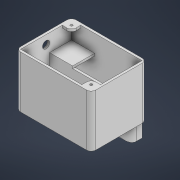
# Autodesk Inventor part: Bike_Telemetry
Saved by Autodesk Inventor 2022 (Build 260153000, 153)
## iProperties
Created: 2022-06-22
Part Number: Bike_Telemetry
Material: Generic
Document SubType Name: Modeling
Designer: Gugarauj07
Density: 1 g/cm^3
Appearance: Default
Author: Gugarauj07
Autodesk Inventor part; units mm, degrees
ref_plane "YZ Plane" through (0, 0, 0) normal (1, 0, 0) x (0, 1, 0)
ref_plane "XZ Plane" through (0, 0, 0) normal (0, 1, 0) x (-1, 0, 0)
ref_plane "XY Plane" through (0, 0, 0) normal (0, 0, 1) x (1, 0, 0)
sketch "Sketch1" plane through (0, 0, 0) normal (0, 0, 1) x (1, 0, 0)
  line L0 (0, 0) -> (65, 0)
  line L1 (65, 0) -> (65, 45)
  line L2 (65, 45) -> (0, 45)
  line L3 (0, 45) -> (0, 0)
  dimension "d3" = 65
  dimension "d4" = 45
  constraints: 8 end point, 2 parallel, 1 horizontal, 1 perpendicular, 1 vertical
  measures "d3" distance of L2.end L1.end
  measures "d4" distance of L1.end L0.end
extrude "Extrusion1" add sketch "Sketch1" along normal blind 48
shell "Shell1" thickness 2 removed faces 1 at (43.3333, 45, 16)
sketch "Sketch2" plane through (2, 2, 2) normal (0, 1, 0) x (1, 0, 0)
  line L0 (61, -44) -> (0, -44) projected
  line L1 (0, -44) -> (10, -44)
  line L2 (10, -44) -> (40, -44)
  line L3 (40, -44) -> (40, -34)
  line L4 (40, -34) -> (10, -34)
  line L5 (10, -34) -> (10, -44)
  line L6 (61, 0) -> (61, -44) projected
  line L7 (0, -44) -> (0, 0) projected
  point P0 (-2, 2)
  dimension "d9" = 30
  dimension "d10" = 10
  dimension "d11" = 61
  dimension "d27" = 10
  constraints: 10 end point, 2 parallel, 1 horizontal, 1 perpendicular, 1 point on line
  measures "d9" distance of L4.end L3.end
  measures "d10" distance of L3.end L2.end
  measures "d11" distance between parallel lines of L6 L7
  measures "d27" distance between parallel lines of L5 L7
extrude "Extrusion2" cut sketch "Sketch2" against normal through all
sketch "Sketch3" plane through (2, 2, 2) normal (0, 1, 0) x (1, 0, 0)
  line L0 (0, 0) -> (0, -44) projected
  line L1 (0, -17) -> (0, 33)
  line L2 (0, -17) -> (44, -17)
  line L3 (44, -17) -> (0, -17)
  line L4 (0, -17) -> (0, -19)
  line L5 (0, -19) -> (44, -19)
  line L6 (44, -19) -> (44, -17)
  point P0 (-2, 2)
  dimension "d16" = 44
  dimension "d17" = 2
  constraints: 12 end point, 2 horizontal, 2 parallel, 2 point on line, 1 collinear, 1 perpendicular
  measures "d16" distance of L1.start L2.end
  measures "d17" distance of L4.end L3.end
extrude "Extrusion3" add sketch "Sketch3" along normal blind 26
fillet "Fillet1" radius 4 1 edges at (0, 22.5, 0)
fillet "Fillet2" radius 4 1 edges at (65, 22.5, 0)
fillet "Fillet3" radius 4 1 edges at (65, 22.5, 48)
fillet "Fillet4" radius 4 1 edges at (0, 22.5, 48)
sketch "Sketch4" plane through (2, 2, 2) normal (1, 0, 0) x (0, 0, -1)
  line L0 (-19, 26) -> (-17, 26) projected
  line L1 (-19, 26) -> (0, 26)
  line L2 (0, 26) -> (0, 28)
  line L3 (0, 28) -> (-19, 28)
  line L4 (-19, 28) -> (-19, 26)
  point P0 (2, -2)
  dimension "d24" = 2
  constraints: 8 end point, 2 parallel, 1 horizontal, 1 perpendicular
  measures "d24" distance of L2.end L1.end
extrude "Extrusion4" add sketch "Sketch4" along normal blind 20
sketch "Sketch8" plane through (2, 2, 2) normal (0, 0, 1) x (1, 0, 0)
  line L0 (0, 43) -> (8, 43)
  line L1 (8, 43) -> (8, 41)
  line L2 (8, 41) -> (0, 41)
  line L3 (0, 41) -> (0, 43)
  point P0 (-2, -2)
  dimension "d28" = 8
  dimension "d29" = 2
  constraints: 8 end point, 2 parallel, 1 horizontal, 1 perpendicular
  measures "d28" distance of L1.end L2.end
  measures "d29" distance of L0.end L1.end
extrude "Extrusion5" add sketch "Sketch8" along normal blind 8
sketch "Sketch10" plane through (4, 45, 0) normal (0, 1, 0) x (1, 0, 0)
  line L0 (6, -2) -> (6, -10) projected
  circle A0 centre (2, -6) radius 1
  point P0 (-4, 0)
  constraints: 1 centre point
extrude "Extrusion7" cut sketch "Sketch10" against normal blind 2
fillet "Fillet6" radius 4 1 edges at (10, 44, 10)
sketch "Sketch13" plane through (63, 45, 46) normal (0, 0, -1) x (-1, 0, 0)
  line L0 (0, -43) -> (0, 0) projected
  line L1 (0, 0) -> (8, 0)
  line L2 (8, 0) -> (8, -2)
  line L3 (8, -2) -> (0, -2)
  line L4 (0, -2) -> (0, 0)
  point P0 (63, -45)
  point P1 (0, -2)
  dimension "d51" = 8
  dimension "d52" = 2
  constraints: 8 end point, 2 parallel, 1 horizontal, 1 perpendicular
  measures "d51" distance of L2.end L3.end
  measures "d52" distance of L1.end L2.end
extrude "Extrusion10" add sketch "Sketch13" along normal blind 8
sketch "Sketch14" plane through (4, 45, 0) normal (0, 1, 0) x (1, 0, 0)
  circle A0 centre (55, -42) radius 1
  point P0 (-4, 0)
  constraints: 1 centre point
extrude "Extrusion11" cut sketch "Sketch14" against normal blind 2
fillet "Fillet7" radius 4 1 edges at (55, 44, 38)
sketch "Sketch15" plane through (4, 0, 0) normal (0, -1, 0) x (1, 0, 0)
  line L0 (57, 0) -> (0, 0)
  line L1 (0, 0) -> (0, 15)
  line L2 (0, 15) -> (57, 15)
  line L3 (57, 15) -> (57, 0)
  constraints: 8 end point, 2 parallel, 1 horizontal, 1 perpendicular
extrude "Extrusion12" add sketch "Sketch15" along normal blind 15
fillet "Fillet8" radius 10 3 edges at (4, -7.5, 15) (61, -7.5, 15) (32.5, -15, 15)
sketch "Sketch16" plane through (0, 0, 0) normal (0, 0, -1) x (-1, 0, 0)
  line L0 (-41, -15) -> (-24, -15)
  line L1 (-24, -15) -> (-24, -10.2203)
  line L2 (-24, -10.2203) -> (-41, -10.2203)
  line L3 (-41, -10.2203) -> (-41, -15)
  point P0 (0, 0)
  point P1 (-4, -15)
  point P2 (-61, -15)
  constraints: 8 end point, 2 parallel, 1 horizontal, 1 perpendicular
extrude "Extrusion13" add sketch "Sketch16" along normal blind 15
fillet "Fillet9" radius 7 2 edges at (41, -12.6102, -15) (24, -12.6102, -15)
sketch "Sketch17" plane through (24, -10.2203, 0) normal (0, 1, 0) x (1, 0, 0)
  line L0 (0, 0) -> (8.5, 0)
  circle A0 centre (8.5, 7.5) radius 4
  point P0 (-24, 0)
  constraints: 2 end point, 1 centre point, 1 horizontal
extrude "Extrusion14" cut sketch "Sketch17" against normal through all
sketch "Sketch19" plane through (2, 2, 46) normal (1, 0, 0) x (0, 0, -1)
  circle A0 centre (22, 35.5) radius 3.125
  point P0 (46, -2)
  point P1 (44, 28)
  dimension "d78" = 6.25
  constraints: 1 centre point
  measures "d78" diameter of A0
extrude "Extrusion15" cut sketch "Sketch19" against normal through all
body "Solid1"
